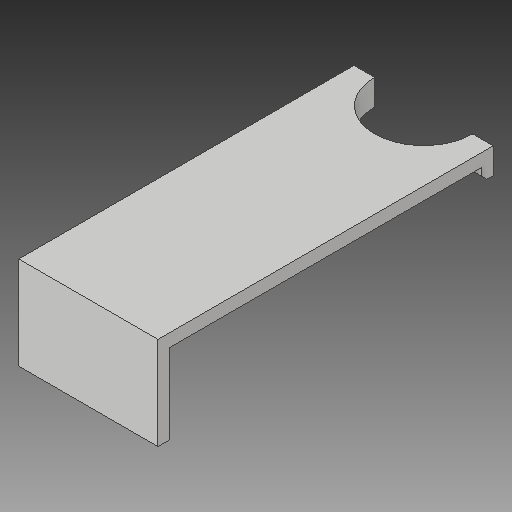
# Autodesk Inventor part: Roof Clip
Saved by Autodesk Inventor 2017 (Build 210142000, 142)
## iProperties
Created: 2018-02-09
Part Number: Roof Clip
Material: Generic
Document SubType Name: Modeling
Designer: Arjuna
Density: 1 g/cm^3
Appearance: Default
Author: Arjuna
Autodesk Inventor part; units mm, degrees
ref_plane "YZ Plane" through (0, 0, 0) normal (1, 0, 0) x (0, 1, 0)
ref_plane "XZ Plane" through (0, 0, 0) normal (0, 1, 0) x (-1, 0, 0)
ref_plane "XY Plane" through (0, 0, 0) normal (0, 0, 1) x (1, 0, 0)
sketch "Sketch3" plane through (0, 0, 0) normal (0, 1, 0) x (-1, 0, 0)
  line L0 (13.5, 0) -> (-13.5, 0)
  line L1 (-13.5, 0) -> (-13.5, -65)
  line L2 (-13.5, -65) -> (13.5, -65)
  line L3 (13.5, -65) -> (13.5, 0)
  point P0 (0, 0)
  dimension "d8" = 27
  dimension "d9" = 13.5
  dimension "d18" = 65
  constraints: 8 end point, 2 parallel, 1 horizontal, 1 perpendicular
  measures "d8" distance of L2.end L1.end
  measures "d9" distance of point (0, 0) L0.start
  measures "d18" distance between parallel lines of L2 L0
extrude "Extrusion3" add sketch "Sketch3" along normal blind 5
sketch "Sketch4" plane through (0, 0, 0) normal (0, -1, 0) x (1, 0, 0)
  line L0 (-13.5, 0) -> (13.5, 0) projected
  line L1 (-13.5, -65) -> (-13.5, 0) projected
  line L2 (13.5, -65) -> (-13.5, -65) projected
  line L3 (13.5, 0) -> (13.5, -65) projected
  line L4 (13.5, 0) -> (-13.5, 0)
  line L5 (-13.5, 0) -> (-13.5, -5)
  line L6 (-13.5, -5) -> (13.5, -5)
  line L7 (13.5, -5) -> (13.5, 0)
  point P0 (0, 0)
  dimension "d14" = 5
  constraints: 8 end point, 2 parallel, 1 horizontal, 1 perpendicular, 1 point on line
  measures "d14" distance between parallel lines of L6 L0
extrude "Extrusion4" add sketch "Sketch4" along normal blind 13 contours L0 L3 L6 L1
sketch "Sketch6" plane through (0, 5, 0) normal (0, 1, 0) x (1, 0, 0)
  line L0 (-13.5, 0) -> (13.5, 0) projected
  line L1 (13.5, 0) -> (13.5, 65) projected
  line L2 (13.5, 65) -> (-13.5, 65) projected
  line L3 (-13.5, 65) -> (-13.5, 0) projected
  circle A0 centre (0, 65) radius 9.5
  point P0 (0, 0)
  dimension "d25" = 19
  dimension "d26" = 0
  constraints: 1 centre point, 1 midpoint
  measures "d25" diameter of A0
  measures "d26" horizontal distance of point (0, 0) A0.centre
extrude "Extrusion6" cut sketch "Sketch6" against normal through all contours A0 L2 | L2 A0
sketch "Sketch7" plane through (13.5, 0, -65) normal (1, 0, 0) x (0, 0, -1)
  line L0 (-60, 0) -> (0, 0) projected
  line L1 (0, 0) -> (0, 5) projected
  line L2 (-65, 5) -> (0, 5) projected
  line L3 (-65, -13) -> (-65, 5) projected
  line L4 (-60, -13) -> (-65, -13) projected
  line L5 (-60, 0) -> (-60, -13) projected
  line L6 (-60, -13) -> (-62.75, -13)
  line L7 (-62.75, -13) -> (-62.75, 0)
  line L8 (-62.75, 0) -> (-60, 0)
  line L9 (-60, 0) -> (-60, -13)
  line L10 (-62.75, 0) -> (-2.25, 0)
  line L11 (-2.25, 0) -> (-2.25, 2.5)
  line L12 (-2.25, 2.5) -> (-62.75, 2.5)
  line L13 (-62.75, 2.5) -> (-62.75, 0)
  point P0 (-65, 0)
  dimension "d29" = 2.75
  dimension "d30" = 2.5
  dimension "d31" = 2.25
  constraints: 16 end point, 4 parallel, 2 horizontal, 2 perpendicular
  measures "d29" distance of L7.end L8.end
  measures "d30" distance between parallel lines of L0 L12
  measures "d31" distance between parallel lines of L1 L11
extrude "Extrusion7" cut sketch "Sketch7" against normal blind 3 contours L8 L13 L12 L11 L0 | L5 L4 L7 L8
mirror "Mirror2" about plane through (0, 0, 0) normal (1, 0, 0) of "Extrusion7"
chamfer "Chamfer1" distance 1 angle 45 2 edges at (12, 0, -62.75) (-12, 0, -62.75)
equation "\"d9\" = 0.5 * d8"
body "Solid2"
